Autodesk Fusion 360 part; units mm, degrees
note: some values were not read from the file. Chosen so that the rebuilt part matches the saved one: which pieces of a blend or face edit are solid.
(part 4 of 5)
  point P179 (230.75, -311.3333)
  point P180 (242.5, -311.3333)
  point P181 (242.5, -311.3333)
  point P182 (219, -320.5)
  point P183 (219, -320.5)
  point P184 (230.75, -320.5)
  point P185 (230.75, -320.5)
  point P186 (242.5, -320.5)
  point P187 (242.5, -320.5)
  point P188 (219, -265.5)
  point P189 (219, -265.5)
  point P190 (230.75, -265.5)
  point P191 (230.75, -265.5)
  point P192 (-15.5, -7.5)
  point P193 (265.5, -242.5)
  point P194 (276.5, -242.5)
  point P195 (265.5, -229.4444)
  point P196 (276.5, -229.4444)
  point P197 (287.5, -242.5)
  point P198 (298.5, -242.5)
  point P199 (309.5, -242.5)
  point P200 (287.5, -229.4444)
  point P201 (298.5, -229.4444)
  point P202 (309.5, -229.4444)
  point P203 (265.5, -216.3889)
  point P204 (276.5, -216.3889)
  point P205 (287.5, -216.3889)
  point P206 (298.5, -216.3889)
  point P207 (309.5, -216.3889)
  point P208 (265.5, -203.3333)
  point P209 (276.5, -203.3333)
  point P210 (287.5, -203.3333)
  point P211 (298.5, -203.3333)
  point P212 (309.5, -203.3333)
  point P213 (265.5, -190.2778)
  point P214 (276.5, -190.2778)
  point P215 (287.5, -190.2778)
  point P216 (298.5, -190.2778)
  point P217 (309.5, -190.2778)
  point P218 (265.5, -177.2222)
  point P219 (265.5, -164.1667)
  point P220 (276.5, -164.1667)
  point P221 (287.5, -164.1667)
  point P222 (298.5, -164.1667)
  point P223 (309.5, -164.1667)
  point P224 (265.5, -151.1111)
  point P225 (276.5, -151.1111)
  point P226 (287.5, -151.1111)
  point P227 (298.5, -151.1111)
  point P228 (309.5, -151.1111)
  point P229 (265.5, -138.0556)
  point P230 (276.5, -138.0556)
  point P231 (287.5, -138.0556)
  point P232 (298.5, -138.0556)
  point P233 (309.5, -138.0556)
  point P234 (265.5, -125)
  point P235 (276.5, -125)
  point P236 (287.5, -125)
  point P237 (298.5, -125)
  point P238 (309.5, -125)
  point P239 (265.5, -111.9444)
  point P240 (276.5, -111.9444)
  point P241 (287.5, -111.9444)
  point P242 (298.5, -111.9444)
  point P243 (309.5, -111.9444)
  point P244 (265.5, -98.8889)
  point P245 (276.5, -98.8889)
  point P246 (287.5, -98.8889)
  point P247 (298.5, -98.8889)
  point P248 (309.5, -98.8889)
  point P249 (265.5, -85.8333)
  point P250 (276.5, -85.8333)
  point P251 (287.5, -85.8333)
  point P252 (298.5, -85.8333)
  point P253 (309.5, -85.8333)
  point P254 (265.5, -72.7778)
  point P255 (276.5, -72.7778)
  point P256 (287.5, -72.7778)
  point P257 (298.5, -72.7778)
  point P258 (309.5, -72.7778)
  point P259 (265.5, -59.7222)
  point P260 (276.5, -59.7222)
  point P261 (287.5, -59.7222)
  point P262 (298.5, -59.7222)
  point P263 (309.5, -59.7222)
  point P264 (265.5, -46.6667)
  point P265 (276.5, -46.6667)
  point P266 (287.5, -46.6667)
  point P267 (298.5, -46.6667)
  point P268 (309.5, -46.6667)
  point P269 (265.5, -33.6111)
  point P270 (276.5, -33.6111)
  point P271 (287.5, -33.6111)
  point P272 (298.5, -33.6111)
  point P273 (309.5, -33.6111)
  point P274 (320.5, -242.5)
  point P275 (320.5, -229.4444)
  point P276 (320.5, -216.3889)
  point P277 (320.5, -203.3333)
  point P278 (320.5, -190.2778)
  point P279 (320.5, -177.2222)
  point P280 (320.5, -164.1667)
  point P281 (320.5, -151.1111)
  point P282 (320.5, -138.0556)
  point P283 (320.5, -125)
  point P284 (320.5, -111.9444)
  point P285 (320.5, -98.8889)
  point P286 (320.5, -85.8333)
  point P287 (320.5, -72.7778)
  point P288 (320.5, -59.7222)
  point P289 (320.5, -46.6667)
  point P290 (320.5, -33.6111)
  point P291 (265.5, -20.5556)
  point P292 (276.5, -20.5556)
  point P293 (287.5, -20.5556)
  point P294 (298.5, -20.5556)
  point P295 (309.5, -20.5556)
  point P296 (320.5, -20.5556)
  point P297 (265.5, -7.5)
  point P298 (276.5, -7.5)
  point P299 (287.5, -7.5)
  point P300 (298.5, -7.5)
  point P301 (309.5, -7.5)
  point P302 (320.5, -7.5)
  point P303 (7.6004, 372.3881)
  point P304 (250, 0)
  point P305 (240, 0)
  point P306 (432.9679, -6)
  point P307 (670.9679, -244)
  dimension "d117" = 241
  dimension "d118" = 241
  dimension "d122" = 235
  dimension "d127" = 4.5
  dimension "d128" = 4.5
  dimension "d179" = 7.5
  dimension "d418" = 8
  dimension "d420" = 11.5
  dimension "d421" = 13
  dimension "d423" = 16.5
  dimension "d425" = 13.5
  dimension "d428" = 7
  dimension "d429" = 15
  dimension "d430" = 7
  dimension "d431" = 13
  dimension "d438" = 8
  dimension "d447" = 17.5
  dimension "d451" = 20
  dimension "d457" = 8
  dimension "d458" = 7.5
  dimension "d461" = 235
  dimension "d517" = 235
  dimension "d521" = 250
  dimension "d522" = 0
  dimension "d531" = 8
  dimension "d532" = 8
  dimension "d533" = 10
  dimension "d534" = 10
  dimension "d537" = 7.5
  dimension "d538" = 7.5
  dimension "d543" = 8
  dimension "d546" = 230
  dimension "d611" = 75
  dimension "d613" = 3.5
  dimension "d614" = 16
  dimension "d616" = 15
  dimension "d617" = 6.5
  dimension "d619" = 15
  dimension "d620" = 1.75
  dimension "d621" = 1.75
  dimension "d622" = 3.75
  dimension "d623" = 3.75
  dimension "d626" = 4.5
  dimension "d627" = 4.5
  dimension "d633" = 235
  dimension "d634" = -55
  dimension "d664" = 6
  dimension "d665" = 12
  dimension "d667" = 4
  dimension "d669" = 6
  dimension "d671" = 4
  dimension "d672" = 2
  dimension "d673" = 24
  dimension "d679" = 12.5
  dimension "d791" = 4.5
  dimension "d792" = 9
  dimension "d793" = 9
  dimension "d796" = 55
  dimension "d797" = 235
  dimension "d802" = 12
  dimension "d808" = 250
  dimension "d822" = 244
  dimension "d823" = 244
  dimension "d898" = 4.5
  dimension "d899" = 3
  dimension "d904" = 3
  dimension "d919" = 0
  dimension "d939" = 3
  dimension "d940" = 3
  dimension "d1030" = 8
  constraint horizontal L3
  constraint vertical L0
  constraint coincident L0.end L3.start
  constraint vertical L1
  constraint vertical L2
  constraint horizontal L5
  constraint horizontal L6
  constraint vertical L7
  constraint coincident P0 A0.centre
  constraint equal A0 A1
  constraint coincident L2.start L8.end
  constraint horizontal L59
  constraint vertical L9
  constraint horizontal L80
  constraint vertical L10
  constraint horizontal L57
  constraint equal L14 L18
  constraint equal L13 L17
  constraint collinear L12 L16
  constraint coincident L32 L33.start
  constraint horizontal L32
  constraint vertical L48
  constraint horizontal L49
  constraint horizontal L50
  constraint vertical L199
  constraint horizontal L51
  constraint collinear L52 L59
  constraint collinear L53 L57
  constraint collinear L54 L59
  constraint collinear L55 L57
  constraint collinear L56 L59
  constraint collinear L57 L58
  constraint collinear L59 L60
  constraint vertical L79
  constraint vertical L62
  constraint horizontal L74
  constraint vertical L73
  constraint horizontal L61
  constraint vertical L72
  constraint horizontal L76
  constraint horizontal L158
  constraint vertical L75
  constraint coincident L75.start L76.end
  constraint equal L77 L78
  constraint horizontal L151
  constraint vertical L70
  constraint horizontal L78
  constraint horizontal L77
  constraint equal L62 L73
  constraint collinear L10 L75
  constraint collinear L48 L72
  constraint collinear L80 L81
  constraint horizontal L84
  constraint vertical L86
  constraint horizontal L85
  constraint vertical L87
  constraint horizontal L89
  constraint vertical L83
  constraint horizontal L82
  constraint vertical L88
  constraint equal A51 A52
  constraint coincident P2 A51.centre
  constraint horizontal L90
  constraint vertical L91
  constraint horizontal L100
  constraint vertical L103
  constraint horizontal L131
  constraint vertical L129
  constraint equal A56 A57
  constraint vertical A56.centre A57.centre
  constraint horizontal L92
  constraint vertical L93
  constraint horizontal L94
  constraint vertical L95
  constraint equal A0 A5
  constraint equal A2 A10
  constraint equal A148 A149
  constraint coincident P192 A148.centre
  constraint collinear L5 L90
  constraint collinear L100 L101
  constraint collinear L102 L129
  constraint collinear L103 L105
  constraint collinear L104 L129
  constraint collinear L105 L107
  constraint collinear L106 L129
  constraint collinear L107 L137
  constraint collinear L108 L129
  constraint coincident L119.start L137
  constraint coincident L117.start L137
  constraint coincident L110.start L137
  constraint coincident L114.start L137
  constraint coincident L112.start L137
  constraint coincident L113.end L131
  constraint coincident L115.end L129
  constraint coincident L116.end L129
  constraint coincident L118.end L129
  constraint coincident L109.end L129
  constraint collinear L126 L129
  constraint collinear L127 L129
  constraint collinear L128 L129
  constraint collinear L129 L130
  constraint collinear L131 L132
  constraint collinear L133 L137
  constraint collinear L134 L137
  constraint collinear L135 L137
  constraint collinear L136 L137
  constraint collinear L137 L138
  constraint equal A153 A154
  constraint coincident P193 A153.centre
  constraint horizontal L142
  constraint vertical L143
  constraint horizontal L144
  constraint vertical L145
  constraint horizontal L146
  constraint vertical L147
  constraint horizontal L148
  constraint vertical L149
  constraint collinear L151 L152
  constraint collinear L152 L153
  constraint collinear L153 L154
  constraint collinear L155 L158
  constraint collinear L156 L158
  constraint collinear L157 L158
  constraint collinear L158 L159
  constraint coincident L50.start L52.end
  constraint coincident P303 A10.centre
  constraint coincident P304 L1.start
  constraint coincident P305 L9.end
  constraint horizontal L160
  constraint vertical L161
  constraint horizontal L162
  constraint vertical L163
  constraint horizontal L164
  constraint vertical L165
  constraint horizontal L166
  constraint vertical L167
  constraint coincident P306 L164.start
  constraint coincident P307 L165.end
  constraint horizontal L171
  constraint vertical L170
  constraint horizontal L173
  constraint vertical L174
  constraint horizontal L175
  constraint vertical L176
  constraint collinear L11 L176
  constraint collinear L37 L174
  constraint collinear L38 L179
  constraint collinear L40 L183
  constraint collinear L43 L186
  constraint collinear L42 L187
  constraint collinear L41 L182
  constraint collinear L39 L178
  constraint collinear L173 L180
  constraint collinear L180 L184
  constraint collinear L184 L188
  constraint equal L176 L179
  constraint equal L176 L178
  constraint equal L176 L182
  constraint equal L176 L183
  constraint equal L176 L187
  constraint equal L176 L186
  constraint equal L75 L79
  constraint collinear L198 L199
  constraint collinear L199 L200
  constraint collinear L200 L201
  constraint collinear L201 L202
  constraint collinear L203 L204
  constraint collinear L204 L205
  constraint collinear L205 L206
  constraint horizontal L211
  constraint vertical L226
  constraint vertical L220
  constraint collinear L220 L222
  constraint collinear L221 L222
  constraint collinear L222 L223
  constraint collinear L224 L226
  constraint collinear L224 L225
  constraint collinear L226 L227
  constraint collinear L227 L228
  measures "d117" distance of L5.start L6.end
  measures "d118" distance of L5.start L5.end
  measures "d127" horizontal distance of L5.start L0.end
  measures "d128" vertical distance of L5.start L0.end
  measures "d179" vertical distance of L4.start A2.centre
  measures "d418" distance of L4.start L11.start
  measures "d420" distance of L28.start L28.end
  measures "d421" distance of L28.start L30.end
  measures "d423" distance of L25.end L26.end
  measures "d425" distance of L24.start L24.end
  measures "d428" distance of L20.end L21.end
  measures "d429" distance of L21.end L22.end
  measures "d430" distance of L16.end L17.end
  measures "d431" distance of L17.end L18.end
  measures "d438" diameter of A3
  measures "d447" distance of L33.start L35.end
  measures "d451" vertical distance of L4.start L32.end
  measures "d457" distance of L50.start L50.end
  measures "d458" horizontal distance of L4.end A2.centre
  measures "d531" distance of L73.start L73.end
  measures "d532" distance of L61.start L61.end
  measures "d533" distance of L61.start L78.start
  measures "d534" distance of L78.start L73.end
  measures "d537" vertical distance of L78.start P303
  measures "d538" horizontal distance of L78.start P303
  measures "d543" distance of L70.start L70.end
  measures "d546" distance of L62.end L73.start
  measures "d613" diameter of A47
  measures "d614" diameter of A48
  measures "d616" vertical distance of A48.centre A46.centre
  measures "d617" diameter of A49
  measures "d619" vertical distance of A47.centre A49.centre
  measures "d620" horizontal distance of A47.centre L84.start
  measures "d621" horizontal distance of L85.start A45.centre
  measures "d622" vertical distance of L85.start A45.centre
  measures "d623" vertical distance of A47.centre L84.start
  measures "d626" horizontal distance of L82.start P1
  measures "d627" vertical distance of L82.start P1
  measures "d664" diameter of A57
  measures "d665" vertical distance of A56.centre A57.centre
  measures "d667" vertical distance of A57.centre P10
  measures "d669" distance of L6 L94
  measures "d671" distance of A57.centre L93
  measures "d672" distance of L93 L95
  measures "d673" distance of L92 L94
  measures "d679" distance of L89 L97
  measures "d791" distance of L91 L99
  measures "d792" distance of L91 L129
  measures "d793" distance of L90 L100
  measures "d802" distance of L146.start L148.end
  measures "d808" distance of L78.start L70.start
  measures "d822" distance of L160.start L160.end
  measures "d823" distance of L160.start L162.end
  measures "d898" distance of L171 L172
  measures "d899" distance of L173.start L175.end
  measures "d904" vertical distance of L64.start L173.start
  measures "d939" distance of L163 L208
  measures "d940" distance of L160 L209
  measures "d1030" distance of L48.start L210.end
sketch "Skizze3" plane through (0, 0, 0) normal (0, 0, 1) x (1, 0, 0)
  circle A0 centre (7.5, -7.5) radius 1.5
  circle A1 centre (7.5, -7.5) radius 1.5
  line L0 (0, 0) -> (15, 0)
  line L1 (15, 0) -> (15, -15)
  line L2 (15, -15) -> (0, -15)
  line L3 (0, -15) -> (0, 0)
  line L4 (15, -15) -> (-13, -15)
  line L5 (-13, -15) -> (-13, 13)
  line L6 (-13, 13) -> (15, 13)
  line L7 (15, 13) -> (15, -15)
  line L8 (15, -15) -> (-8, -15)
  line L9 (-8, -15) -> (-8, 8)
  line L10 (-8, 8) -> (15, 8)
  line L11 (15, 8) -> (15, -15)
  line L12 (-8, -15) -> (-11, -15)
  line L13 (-11, -15) -> (-11, -4.5)
  line L14 (-11, -4.5) -> (-8, -4.5)
  line L15 (-8, -4.5) -> (-8, -15)
  line L16 (15, 8) -> (4.5, 8)
  line L17 (4.5, 11) -> (15, 11)
  line L18 (15, 11) -> (15, 8)
  line L19 (0, 0) -> (10.8258, 0)
  line L20 (10.8258, 0) -> (10.8258, 2.5)
  line L21 (10.8258, 2.5) -> (0, 2.5)
  line L22 (0, 2.5) -> (0, 0)
  line L23 (0, 2.5) -> (15, 2.5)
  line L24 (15, 2.5) -> (15, 5.5)
  line L25 (15, 5.5) -> (0, 5.5)
  line L26 (0, 5.5) -> (0, 2.5)
  line L27 (29.799, -19.957) -> (29.799, -30.0096)
  line L28 (24.9821, -24.9833) -> (34.8253, -24.9833)
  line L29 (4.5, -4.5) -> (15, -4.5)
  line L30 (15, -4.5) -> (15, -15)
  line L31 (15, -15) -> (4.5, -15)
  line L32 (4.5, -15) -> (4.5, -4.5)
  line L33 (4.5, 8) -> (4.5, 11)
  line L34 (4.5, -4.5) -> (245.5, -4.5)
  line L35 (0, 5.5) -> (0, 8)
  line L36 (44.598, -15) -> (59.598, -15)
  line L37 (59.598, 2.5) -> (44.598, 2.5)
  line L38 (48.7722, 0) -> (48.7722, 2.5)
  line L39 (59.598, -15) -> (59.598, 0)
  line L40 (59.598, 0) -> (48.7722, 0)
  line L41 (67.598, -4.5) -> (67.598, -15)
  line L42 (72.598, 13) -> (44.598, 13)
  line L43 (55.098, 11) -> (44.598, 11)
  line L44 (72.598, -15) -> (72.598, 13)
  line L45 (67.598, -15) -> (70.598, -15)
  line L46 (59.598, 5.5) -> (59.598, 8)
  line L47 (44.598, 5.5) -> (59.598, 5.5)
  line L48 (44.598, 0) -> (44.598, -15)
  line L49 (55.098, 8) -> (55.098, 11)
  line L50 (44.598, 8) -> (44.598, -15)
  line L51 (70.598, -4.5) -> (67.598, -4.5)
  line L52 (44.598, -15) -> (67.598, -15)
  line L53 (67.598, 8) -> (44.598, 8)
  circle A2 centre (52.098, -7.5) radius 1.5
  line L54 (44.598, -15) -> (55.098, -15)
  line L55 (67.598, -15) -> (67.598, 8)
  line L56 (44.598, 11) -> (44.598, 8)
  line L57 (44.598, -4.5) -> (44.598, -15)
  line L58 (44.598, 2.5) -> (44.598, 5.5)
  line L59 (59.598, 2.5) -> (59.598, 0)
  circle A3 centre (52.098, -7.5) radius 1.5
  line L60 (70.598, -15) -> (70.598, -4.5)
  line L61 (55.098, -15) -> (55.098, -4.5)
  line L62 (59.598, 5.5) -> (59.598, 2.5)
  line L63 (55.098, -4.5) -> (44.598, -4.5)
  line L64 (44.598, -15) -> (72.598, -15)
  line L65 (48.7722, 2.5) -> (59.598, 2.5)
  line L66 (59.598, 0) -> (44.598, 0)
  line L67 (44.598, 8) -> (55.098, 8)
  line L68 (44.598, 13) -> (44.598, -15)
  line L69 (15, -52.4665) -> (15, -55.4665)
  line L70 (44.598, -49.9665) -> (44.598, -34.9665)
  line L71 (48.7722, -49.9665) -> (48.7722, -52.4665)
  circle A4 centre (52.098, -42.4665) radius 1.5
  line L72 (44.598, -45.4665) -> (44.598, -34.9665)
  circle A5 centre (52.098, -42.4665) radius 1.5
  line L73 (59.598, -49.9665) -> (44.598, -49.9665)
  line L74 (59.598, -52.4665) -> (44.598, -52.4665)
  line L75 (44.598, -34.9665) -> (59.598, -34.9665)
  line L76 (44.598, -34.9665) -> (67.598, -34.9665)
  line L77 (55.098, -60.9665) -> (44.598, -60.9665)
  line L78 (55.098, -45.4665) -> (44.598, -45.4665)
  line L79 (67.598, -57.9665) -> (44.598, -57.9665)
  line L80 (59.598, -49.9665) -> (48.7722, -49.9665)
  line L81 (48.7722, -52.4665) -> (59.598, -52.4665)
  line L82 (44.598, -34.9665) -> (72.598, -34.9665)
  line L83 (72.598, -62.9665) -> (44.598, -62.9665)
  line L84 (44.598, -57.9665) -> (55.098, -57.9665)
  line L85 (44.598, -55.4665) -> (59.598, -55.4665)
  line L86 (44.598, -34.9665) -> (55.098, -34.9665)
  line L87 (15, -45.4665) -> (15, -34.9665)
  line L88 (4.5, -34.9665) -> (4.5, -45.4665)
  line L89 (15, -57.9665) -> (15, -34.9665)
  line L90 (-8, -34.9665) -> (-8, -57.9665)
  line L91 (-8, -57.9665) -> (15, -57.9665)
  line L92 (44.598, -62.9665) -> (44.598, -34.9665)
  line L93 (10.8258, -52.4665) -> (0, -52.4665)
  line L94 (0, -55.4665) -> (0, -57.9665)
  line L95 (15, -57.9665) -> (4.5, -57.9665)
  line L96 (0, -52.4665) -> (15, -52.4665)
  line L97 (0, -49.9665) -> (10.8258, -49.9665)
  line L98 (44.598, -60.9665) -> (44.598, -57.9665)
  line L99 (15, -62.9665) -> (15, -34.9665)
  line L100 (44.598, -52.4665) -> (44.598, -55.4665)
  line L101 (15, -34.9665) -> (0, -34.9665)
  line L102 (15, -60.9665) -> (15, -57.9665)
  line L103 (-13, -34.9665) -> (-13, -62.9665)
  circle A6 centre (7.5, -42.4665) radius 1.5
  line L104 (-11, -45.4665) -> (-8, -45.4665)
  line L105 (0, -49.9665) -> (15, -49.9665)
  line L106 (4.5, -57.9665) -> (4.5, -60.9665)
  line L107 (44.598, -57.9665) -> (44.598, -34.9665)
  line L108 (0, -52.4665) -> (0, -49.9665)
  line L109 (0, -34.9665) -> (0, -49.9665)
  line L110 (10.8258, -49.9665) -> (10.8258, -52.4665)
  line L111 (0, -55.4665) -> (0, -52.4665)
  circle A7 centre (7.5, -42.4665) radius 1.5
  line L112 (4.5, -45.4665) -> (15, -45.4665)
  line L113 (15, -34.9665) -> (-13, -34.9665)
  line L114 (15, -49.9665) -> (15, -34.9665)
  line L115 (15, -34.9665) -> (4.5, -34.9665)
  line L116 (15, -55.4665) -> (0, -55.4665)
  line L117 (4.5, -60.9665) -> (15, -60.9665)
  line L118 (-8, -34.9665) -> (-11, -34.9665)
  line L119 (-13, -62.9665) -> (15, -62.9665)
  line L120 (-8, -45.4665) -> (-8, -34.9665)
  line L121 (-11, -34.9665) -> (-11, -45.4665)
  line L122 (15, -34.9665) -> (-8, -34.9665)
  line L123 (59.598, -52.4665) -> (59.598, -49.9665)
  line L124 (59.598, -55.4665) -> (59.598, -57.9665)
  line L125 (70.598, -34.9665) -> (70.598, -45.4665)
  line L126 (67.598, -34.9665) -> (67.598, -57.9665)
  line L127 (67.598, -45.4665) -> (67.598, -34.9665)
  line L128 (59.598, -55.4665) -> (59.598, -52.4665)
  line L129 (59.598, -34.9665) -> (59.598, -49.9665)
  line L130 (55.098, -57.9665) -> (55.098, -60.9665)
  line L131 (55.098, -34.9665) -> (55.098, -45.4665)
  line L132 (70.598, -45.4665) -> (67.598, -45.4665)
  line L133 (72.598, -34.9665) -> (72.598, -62.9665)
  line L134 (67.598, -34.9665) -> (70.598, -34.9665)
  point P0 (7.5, -7.5)
  point P1 (4.5, -4.5)
  point P2 (59.598, 0)
  point P3 (52.098, -7.5)
  point P4 (55.098, -4.5)
  point P5 (55.098, -4.5)
  point P6 (7.5, -42.4665)
  point P7 (55.098, -45.4665)
  point P8 (52.098, -42.4665)
  point P9 (55.098, -45.4665)
  point P10 (0, -49.9665)
  point P11 (59.598, -49.9665)
  point P12 (4.5, -45.4665)
  point P13 (4.5, -45.4665)
  dimension "d971" = 15
  dimension "d972" = 15
  dimension "d973" = 28
  dimension "d974" = 28
  dimension "d975" = 23
  dimension "d976" = 23
  dimension "d977" = 3
  dimension "d980" = 3
  dimension "d981" = 2.5
  dimension "d982" = 3
  constraint coincident P0 A0.centre
  constraint equal A0 A1
  constraint horizontal L0
  constraint vertical L1
  constraint horizontal L2
  constraint vertical L3
  constraint coincident L0.start L3.end
  constraint horizontal L4
  constraint vertical L5
  constraint horizontal L6
  constraint vertical L7
  constraint horizontal L8
  constraint vertical L9
  constraint horizontal L10
  constraint vertical L11
  constraint horizontal L12
  constraint vertical L13
  constraint horizontal L14
  constraint vertical L15
  constraint horizontal L16
  constraint horizontal L17
  constraint vertical L18
  constraint horizontal L19
  constraint vertical L20
  constraint horizontal L21
  constraint vertical L22
  constraint horizontal L23
  constraint vertical L24
  constraint horizontal L25
  constraint vertical L26
  constraint coincident L7 L24.end
  constraint vertical L27
  constraint perpendicular L27 L28
  constraint horizontal L29
  constraint vertical L30
  constraint horizontal L31
  constraint vertical L32
  constraint coincident P1 L29.start
  constraint perpendicular L17 L33
  constraint collinear L32 L33
  constraint collinear L14 L34
  constraint coincident L10 L35.end
  constraint perpendicular L10 L35
  constraint symmetric L0.start L27 P2
  constraint symmetric A0 L27 A2
  constraint symmetric P0 L27 P3
  constraint symmetric A1 L27 A3
  constraint symmetric L0.end L27 L48.start
  constraint symmetric L1.end L27 L36.start
  constraint symmetric L2.end L27 L36.end
  constraint symmetric L4.end L27 L44.start
  constraint symmetric L5.end L27 L42.start
  constraint symmetric L6.end L27 L42.end
  constraint symmetric L8.end L27 L41.end
  constraint symmetric L9.end L27 L53.start
  constraint symmetric L10.end L27 L50.start
  constraint symmetric L12.end L27 L45.end
  constraint symmetric L13.end L27 L51.start
  constraint symmetric L14.end L27 L41.start
  constraint symmetric L16.end L27 L49.start
  constraint symmetric L17.start L27 L43.start
  constraint symmetric L17.end L27 L43.end
  constraint symmetric L19.end L27 L38.start
  constraint symmetric L20.end L27 L38.end
  constraint symmetric L21.end L27 L37.start
  constraint symmetric L23.end L27 L37.end
  constraint symmetric L24.end L27 L47.start
  constraint symmetric L25.end L27 L46.start
  constraint symmetric L27 P1 P5
  constraint symmetric L27 L29.end L57.start
  constraint symmetric L27 L31.end L54.end
  constraint symmetric L27 L35.end L46.end
  constraint symmetric L0.start L28 P10
  constraint symmetric A0 L28 A7
  constraint symmetric P0 L28 P6
  constraint symmetric A1 L28 A6
  constraint symmetric L0.end L28 L105.end
  constraint symmetric L1.end L28 L87.end
  constraint symmetric L2.end L28 L101.end
  constraint symmetric L4.end L28 L103.start
  constraint symmetric L5.end L28 L103.end
  constraint symmetric L6.end L28 L99.start
  constraint symmetric L8.end L28 L90.start
  constraint symmetric L9.end L28 L90.end
  constraint symmetric L10.end L28 L89.start
  constraint symmetric L12.end L28 L118.end
  constraint symmetric L13.end L28 L104.start
  constraint symmetric L14.end L28 L104.end
  constraint symmetric L16.end L28 L95.end
  constraint symmetric L17.start L28 L106.end
  constraint symmetric L17.end L28 L102.start
  constraint symmetric L19.end L28 L97.end
  constraint symmetric L20.end L28 L93.start
  constraint symmetric L21.end L28 L93.end
  constraint symmetric L23.end L28 L69.start
  constraint symmetric L24.end L28 L69.end
  constraint symmetric L25.end L28 L94.start
  constraint symmetric L28 P1 P13
  constraint symmetric L28 L29.end L87.start
  constraint symmetric L28 L31.end L88.start
  constraint symmetric L28 L35.end L94.end
  constraint symmetric L28 L37.start L74.start
  constraint symmetric L28 L36.end L75.end
  constraint symmetric L28 L41.end L76.end
  constraint symmetric L28 L54.end L86.end
  constraint symmetric L28 L38.start L71.start
  constraint symmetric L28 L46.start L85.end
  constraint symmetric L28 L48.start L70.start
  constraint symmetric L28 L46.end L124.end
  constraint symmetric L28 L36.start L70.end
  constraint symmetric L28 L42.start L83.start
  constraint symmetric L28 P2 P11
  constraint symmetric L28 L50.start L79.end
  constraint symmetric L28 L42.end L83.end
  constraint symmetric L28 L45.end L125.start
  constraint symmetric L28 P3 P8
  constraint symmetric L28 L57.start L72.start
  constraint symmetric L28 L41.start L127.start
  constraint symmetric L28 P5 P9
  constraint symmetric L28 L51.start L125.end
  constraint symmetric L28 L49.start L84.end
  constraint symmetric L28 L43.start L77.start
  constraint symmetric L28 L37.end L74.end
  constraint symmetric L28 L53.start L79.start
  constraint symmetric L28 L47.start L85.start
  constraint symmetric L28 L44.start L82.end
  constraint symmetric L28 L38.end L71.end
  constraint symmetric L28 L43.end L77.end
  constraint symmetric L28 A2 A5
  constraint symmetric L28 A3 A4
  measures "d971" distance of L0.start L0.end
  measures "d972" distance of L0.start L2.end
  measures "d973" distance of L1.end L4.end
  measures "d974" distance of L1.end L6.end
  measures "d975" distance of L1.end L8.end
  measures "d976" distance of L1.end L10.end
  measures "d977" distance of L8.end L12.end
  measures "d980" distance of L10.end L17.end
  measures "d981" distance of L0.start L21.end
  measures "d982" distance of L21.end L25.end
sketch "Skizze4" plane through (-10, 0, 0) normal (-1, 0, 0) x (0, -1, 0)
  line L0 (-10, 0) -> (-8, 0)
  line L1 (15, 70) -> (15, 75)
  line L2 (15, 75) -> (-10, 75)
  line L3 (-10, 75) -> (-10, 0)
  circle A0 centre (7.5, 62.5) radius 1.5
  circle A1 centre (7.5, 7.5) radius 1.5
  line L4 (-8, 70) -> (15, 70)
  line L5 (-8, 0) -> (-8, 70)
  point P0 (-10, 0)
  dimension "d167" = 3
  dimension "d168" = 17.5
  dimension "d169" = 12.5
  dimension "d337" = 3
  dimension "d338" = 17.5
  dimension "d339" = 7.5
  measures "d167" diameter of A0
  measures "d168" horizontal distance of L2.end A0.centre
  measures "d169" vertical distance of L2.end A0.centre
  measures "d337" diameter of A1
  measures "d338" horizontal distance of A1.centre P0
  measures "d339" vertical distance of A1.centre origin
sketch "Skizze5" plane through (0, 0, 0) normal (0, 0, 1) x (1, 0, 0)
  line L0 (0, 7.8901) -> (0, 0)
  line L1 (15, 20) -> (40, 20)
  line L2 (40, 20) -> (40, 45)
  line L3 (40, 45) -> (15, 45)
  line L4 (15, 45) -> (15, 20)
  line L5 (40, 45) -> (17, 45)
  line L6 (17, 45) -> (17, 22)
  line L7 (17, 22) -> (40, 22)
  line L8 (40, 22) -> (40, 45)
  circle A0 centre (32.5, 37.5) radius 1.5
  dimension "d207" = 25
  dimension "d208" = 23
  dimension "d209" = 3
  dimension "d210" = 7.5
  dimension "d211" = 7.5
  constraint horizontal L1
  constraint vertical L2
  constraint horizontal L3
  constraint vertical L4
  constraint equal L1 L4
  constraint horizontal L5
  constraint vertical L6
  constraint horizontal L7
  constraint vertical L8
  constraint equal L5 L8
  measures "d207" distance of L1.start L3.end
  measures "d208" distance of L2.end L7.end
  measures "d209" diameter of A0
  measures "d210" horizontal distance of L2.end A0.centre
  measures "d211" vertical distance of L2.end A0.centre
sketch "Skizze6" plane through (0, 0, 0) normal (0, 0, 1) x (1, 0, 0)
  line L0 (45.0336, 39.9327) -> (60.0336, 39.9327)
  line L1 (60.0336, 39.9327) -> (60.0336, 24.9327)
  line L2 (60.0336, 24.9327) -> (45.0336, 24.9327)
  line L3 (45.0336, 24.9327) -> (45.0336, 39.9327)
  line L4 (60.0336, 39.9327) -> (47.0336, 39.9327)
  line L5 (47.0336, 39.9327) -> (47.0336, 26.9327)
  line L6 (47.0336, 26.9327) -> (60.0336, 26.9327)
  line L7 (60.0336, 26.9327) -> (60.0336, 39.9327)
  circle A0 centre (52.5336, 32.4327) radius 1.5
  dimension "d213" = 15
  dimension "d214" = 13
  dimension "d243" = 3
  dimension "d244" = 7.5
  dimension "d245" = 7.5
  constraint horizontal L0
  constraint vertical L1
  constraint horizontal L2
  constraint vertical L3
  constraint equal L0 L3
  constraint horizontal L4
  constraint vertical L5
  constraint horizontal L6
  constraint vertical L7
  constraint equal L5 L6
  measures "d213" distance of L0.start L2.end
  measures "d214" distance of L0.end L6.end
  measures "d243" diameter of A0
  measures "d244" horizontal distance of L0.end A0.centre
  measures "d245" vertical distance of L0.end A0.centre
extrude "Extrusion7" add sketch "Skizze5" along normal blind 2 contours L2 L3 L5 L6 L7 L8 makes body 1
extrude "Extrusion8" add sketch "Skizze6" along normal blind 2 separate body contours L0 L1 L4 L5 L6 L7 | A0 makes body 2
extrude "Extrusion9" add sketch "Skizze5" along normal blind 25 contours L1 L2 L3 L4 L6 L7 bodies 1
extrude "Extrusion10" add sketch "Skizze6" along normal blind 15 contours L0 L1 L2 L3 L5 L6 bodies 2
sketch "Skizze7" plane through (0, 24.9327, 0) normal (0, -1, 0) x (1, 0, 0)
  line L0 (45.0336, 0) -> (60.0336, 0)
  line L1 (60.0336, 0) -> (60.0336, 15)
  line L2 (60.0336, 15) -> (45.0336, 15)
  line L3 (45.0336, 15) -> (45.0336, 0)
  circle A0 centre (52.5336, 7.5) radius 1.5
  dimension "d223" = 3
  dimension "d224" = 7.5
  dimension "d225" = 7.5
  measures "d223" diameter of A0
  measures "d224" horizontal distance of L1.end A0.centre
  measures "d225" vertical distance of L1.end A0.centre
sketch "Skizze8" plane through (0, 20, 0) normal (0, -1, 0) x (1, 0, 0)
  line L0 (15, 0) -> (40, 0)
  line L1 (40, 0) -> (40, 25)
  line L2 (40, 25) -> (15, 25)
  line L3 (15, 25) -> (15, 0)
  circle A0 centre (32.5, 17.5) radius 1.5
  dimension "d226" = 3
  dimension "d227" = 7.5
  dimension "d228" = 7.5
  measures "d226" diameter of A0
  measures "d227" horizontal distance of L1.end A0.centre
  measures "d228" vertical distance of L1.end A0.centre
sketch "Skizze9" plane through (15, 0, 0) normal (-1, 0, 0) x (0, -1, 0)
  line L0 (-45, 0) -> (-20, 0)
  line L1 (-20, 0) -> (-20, 25)
  line L2 (-20, 25) -> (-45, 25)
  line L3 (-45, 25) -> (-45, 0)
  circle A0 centre (-37.5, 17.5) radius 1.5
  dimension "d229" = 3
  dimension "d230" = 7.5
  dimension "d231" = 7.5
  measures "d229" diameter of A0
  measures "d230" vertical distance of L2.end A0.centre
  measures "d231" horizontal distance of L2.end A0.centre
sketch "Skizze10" plane through (45.0336, 0, 0) normal (-1, 0, 0) x (0, -1, 0)
  line L0 (-39.9327, 0) -> (-24.9327, 0)
  line L1 (-24.9327, 0) -> (-24.9327, 15)
  line L2 (-24.9327, 15) -> (-39.9327, 15)
  line L3 (-39.9327, 15) -> (-39.9327, 0)
  circle A0 centre (-32.4327, 7.5) radius 1.5
  dimension "d232" = 3
  dimension "d233" = 7.5
  dimension "d234" = 7.5
  measures "d232" diameter of A0
  measures "d233" horizontal distance of L2.end A0.centre
  measures "d234" vertical distance of L2.end A0.centre
extrude "Extrusion11" cut sketch "Skizze8" against normal blind 2 contours A0 bodies 1
extrude "Extrusion12" cut sketch "Skizze9" against normal blind 2 contours A0 bodies 1
extrude "Extrusion13" cut sketch "Skizze7" against normal blind 2 contours A0 bodies 2
extrude "Extrusion14" cut sketch "Skizze10" against normal blind 2 contours A0 bodies 2
extrude "Extrusion15" cut sketch "Skizze6" along normal blind 2 contours A0 bodies 2
sketch "Skizze11" plane through (0, 0, 0) normal (0, 0, 1) x (1, 0, 0)
  line L0 (15, 50) -> (40, 50)
  line L1 (40, 50) -> (40, 65)
  line L2 (40, 65) -> (15, 65)
  line L3 (15, 65) -> (15, 50)
  line L4 (40, 65) -> (17, 65)
  line L5 (17, 65) -> (17, 50)
  line L6 (17, 50) -> (40, 50)
  line L7 (40, 50) -> (40, 65)
  circle A0 centre (32.5, 57.5) radius 1.5
  line L8 (40, 116) -> (15, 116)
  line L9 (40, 75) -> (40, 116)
  line L10 (17, 116) -> (17, 75)
  line L11 (40, 75) -> (40, 116)
  line L12 (17, 75) -> (40, 75)
  line L13 (40, 116) -> (17, 116)
  line L14 (15, 75) -> (40, 75)
  line L15 (15, 116) -> (15, 75)
  circle A1 centre (32.5, 108.5) radius 1.5
  circle A2 centre (32.5, 82.5) radius 1.5
  dimension "d301" = 25
  dimension "d302" = 15
  dimension "d303" = 23
  dimension "d304" = 3
  dimension "d305" = 7.5
  dimension "d306" = 7.5
  dimension "d1009" = 25
  dimension "d1010" = 41
  dimension "d1011" = 23
  dimension "d1012" = 3
  dimension "d1013" = 7.5
  dimension "d1014" = 7.5
  dimension "d1015" = 3
  dimension "d1016" = 7.5
  dimension "d1017" = 7.5
  constraint horizontal L0
  constraint vertical L1
  constraint horizontal L2
  constraint vertical L3
  constraint horizontal L4
  constraint vertical L5
  constraint horizontal L6
  constraint vertical L7
  constraint horizontal L14
  constraint vertical L9
  constraint horizontal L8
  constraint vertical L15
  constraint horizontal L13
  constraint vertical L10
  constraint horizontal L12
  constraint vertical L11
  measures "d301" distance of L0.start L0.end
  measures "d302" distance of L0.start L2.end
  measures "d303" distance of L1.end L4.end
  measures "d304" diameter of A0
  measures "d305" horizontal distance of L1.end A0.centre
  measures "d306" vertical distance of L1.end A0.centre
  measures "d1009" distance of L14.start L9.start
  measures "d1010" distance of L14.start L8.end
  measures "d1011" distance of L8.start L10.start
  measures "d1012" diameter of A1
  measures "d1013" horizontal distance of L8.start A1.centre
  measures "d1014" vertical distance of L8.start A1.centre
  measures "d1015" diameter of A2
  measures "d1016" distance of L11 A2.centre
  measures "d1017" distance of L14 A2.centre
extrude "Extrusion16" add sketch "Skizze11" along normal blind 2 separate body contours L0 L1 L2 L4 L5 L6 L7 | L8 L9 L10 L11 L12 L13 L14 makes body 3 at (21.6667, 57.5, 0) makes body 4 at (21.7535, 91.4483, 0)
extrude "Extrusion17" add sketch "Skizze11" along normal blind 25 contours L0 L2 L3 L5 | L8 L10 L14 L15 bodies 3 4
sketch "Skizze12" plane through (15, 0, 0) normal (-1, 0, 0) x (0, -1, 0)
  line L0 (-65, 0) -> (-50, 0)
  line L1 (-50, 0) -> (-50, 25)
  line L2 (-50, 25) -> (-65, 25)
  line L3 (-65, 25) -> (-65, 0)
  circle A0 centre (-57.5, 17.5) radius 1.5
  circle A1 centre (-108.5, 17.5) radius 1.5
  circle A2 centre (-82.5, 17.5) radius 1.5
  line L4 (-75, 0) -> (-75, 25)
  line L5 (-116, 0) -> (-116, 25)
  line L6 (-116, 25) -> (-75, 25)
  dimension "d311" = 3
  dimension "d312" = 7.5
  dimension "d313" = 7.5
  dimension "d1018" = 3
  dimension "d1019" = 3
  dimension "d1020" = 7.5
  dimension "d1021" = 7.5
  dimension "d1022" = 7.5
  dimension "d1023" = 7.5
  measures "d311" diameter of A0
  measures "d312" horizontal distance of L2.end A0.centre
  measures "d313" vertical distance of L2.end A0.centre
  measures "d1018" diameter of A1
  measures "d1019" diameter of A2
  measures "d1020" distance of A2.centre L4
  measures "d1021" distance of A1.centre L5
  measures "d1022" distance of A1.centre L6
  measures "d1023" distance of A2.centre L6
sketch "Skizze13" plane through (0, 0, 0) normal (0, 0, 1) x (1, 0, 0)
  line L0 (45.0336, 49.7292) -> (60.0336, 49.7292)
  line L1 (60.0336, 49.7292) -> (60.0336, 64.7292)
  line L2 (60.0336, 64.7292) -> (45.0336, 64.7292)
  line L3 (45.0336, 64.7292) -> (45.0336, 49.7292)
  circle A0 centre (52.5336, 57.2292) radius 1.5
  line L4 (60.0336, 64.7292) -> (47.0336, 64.7292)
  line L5 (47.0336, 64.7292) -> (47.0336, 49.7292)
  line L6 (47.0336, 49.7292) -> (60.0336, 49.7292)
  line L7 (60.0336, 49.7292) -> (60.0336, 64.7292)
  line L8 (47.0336, 62.7292) -> (60.0336, 62.7292)
  line L9 (60.0336, 62.7292) -> (60.0336, 51.7292)
  line L10 (60.0336, 51.7292) -> (47.0336, 51.7292)
  line L11 (47.0336, 51.7292) -> (47.0336, 62.7292)
  dimension "d314" = 15
  dimension "d315" = 15
  dimension "d316" = 3
  dimension "d317" = 7.5
  dimension "d318" = 7.5
  dimension "d319" = 13
  dimension "d320" = 15
  dimension "d321" = 13
  dimension "d322" = 11
  dimension "d323" = 2
  constraint horizontal L0
  constraint vertical L1
  constraint horizontal L2
  constraint vertical L3
  constraint horizontal L4
  constraint vertical L5
  constraint horizontal L6
  constraint vertical L7
  constraint horizontal L8
  constraint vertical L9
  constraint horizontal L10
  constraint vertical L11
  constraint coincident L5 L8.start
  measures "d314" distance of L0.start L0.end
  measures "d315" distance of L0.start L2.end
  measures "d316" diameter of A0
  measures "d317" horizontal distance of L1.end A0.centre
  measures "d318" vertical distance of L1.end A0.centre
  measures "d319" distance of L1.end L4.end
  measures "d320" distance of L1.end L0.end
  measures "d321" distance of L8.start L8.end
  measures "d322" distance of L8.start L10.end
  measures "d323" distance of L4.end L8.start
extrude "Extrusion18" add sketch "Skizze13" along normal blind 2 separate body contours L1 L5 L7 L8 L9 L10 L11 makes body 5
extrude "Extrusion19" add sketch "Skizze13" along normal blind 15 contours L0 L1 L5 L6 L7 L10 | L1 L2 L4 L5 L7 L8 bodies 5
extrude "Extrusion20" add sketch "Skizze13" along normal blind 15 contours L0 L2 L3 L5 L11 bodies 5
draft "Entwurf1" angle -45 neutral plane through (45.0336, 64.7292, 0) pull (-1, 0, 0) 1 faces at (50.7003, 50.3959, 15) on bodies 5
sketch "Skizze14" plane through (45.0336, 0, 0) normal (-1, 0, 0) x (0, -1, 0)
  line L0 (-64.7292, 0) -> (-49.7292, 0)
  line L1 (-49.7292, 0) -> (-49.7292, 15)
  line L2 (-49.7292, 15) -> (-64.7292, 15)
  line L3 (-64.7292, 15) -> (-64.7292, 0)
  circle A0 centre (-57.2292, 7.5) radius 1.5
  dimension "d332" = 3
  dimension "d333" = 7.5
  dimension "d334" = 7.5
  measures "d332" diameter of A0
  measures "d333" horizontal distance of L2.end A0.centre
  measures "d334" vertical distance of L2.end A0.centre
extrude "Extrusion21" cut sketch "Skizze14" against normal blind 2 contours A0 bodies 5
extrude "Extrusion23" cut sketch "Skizze12" against normal blind 2 contours A0 | A1 | A2 bodies 3 4
extrude "Extrusion24" add sketch "Skizze3" along normal blind 5 separate body contours L0 L19 L20 L21 L22 L23 | L0 L1 L2 L3 L4 L7 L8 L11 L19 L29 L32 L34 | L3 L4 L8 L9 L10 L15 L22 L26 L35 | L0 L7 L11 L20 L23 | L7 L11 L21 L23 L24 L25 L26 | L4 L9 L12 L13 L14 L15 | L7 L10 L11 L16 L25 L35 | L4 L5 L6 L7 L9 L10 L13 L14 L17 L33 | L7 L10 L16 L17 L18 L33 | L34 L39 L40 L48 L50 L63 L66 L68 | L34 L36 L39 L52 L61 L64 | L37 L38 L50 L66 L68 | L34 L39 L46 L53 L55 L59 L62 | L34 L39 L41 L52 L55 L64 | L37 L47 L50 L58 L62 L65 L68 | L37 L38 L40 L59 L65 L66 | L34 L42 L43 L44 L49 L51 L53 L55 L68 | L34 L41 L45 L51 L55 L60 L64 | L46 L47 L50 L53 L67 L68 | L34 L44 L60 L64 | L43 L49 L53 L56 L67 L68 | L89 L96 L99 L105 L110 | L69 L89 L93 L96 L99 L111 L116 | L89 L91 L94 L95 L99 L116 | L88 L89 L97 L99 L101 L105 L109 L112 L113 L114 L122 | L93 L96 L97 L105 L108 L110 | L91 L95 L99 L102 L106 L117 | L90 L91 L94 L108 L109 L111 L113 L120 L122 | L90 L91 L99 L103 L104 L106 L113 L117 L119 L121 | L90 L104 L113 L118 L120 L121 | L70 L73 L75 L76 L78 L80 L82 L92 L107 L129 L131 | L71 L73 L74 L92 L107 | L71 L73 L74 L80 L81 L123 | L74 L81 L85 L92 L100 L107 L128 | L76 L79 L82 L123 L124 L126 L127 L128 L129 | L79 L84 L85 L92 L107 L124 | L77 L79 L84 L92 L98 L130 | L82 L125 L126 L127 L132 L134 | L77 L79 L82 L83 L92 L125 L126 L130 L132 L133 makes body 6 at (-7.1667, -2.1667, 0) makes body 7 at (-7.1667, -47.7999, 5) makes body 8 at (57.4313, -57.1332, 5) makes body 9 at (57.4313, 7.1667, 0)
extrude "Extrusion32" add sketch "Skizze3" along normal blind 2 contours L1 L2 L4 L7 L8 L11 L29 L30 L31 L32 L34 | L34 L36 L48 L50 L52 L54 L57 L61 L63 L64 L68 | L87 L88 L89 L99 L101 L112 L113 L114 L115 L122 | L70 L72 L75 L76 L78 L82 L86 L92 L107 L131 bodies 7 8 6 9
extrude "Extrusion33" add sketch "Skizze3" along normal blind 28 contours L7 L10 L11 L16 L25 L35 | L4 L5 L6 L7 L9 L10 L13 L14 L17 L33 | L7 L10 L16 L17 L18 L33 | L34 L42 L43 L44 L49 L51 L53 L55 L68 | L46 L47 L50 L53 L67 L68 | L34 L44 L60 L64 | L43 L49 L53 L56 L67 L68 | L90 L91 L99 L103 L104 L106 L113 L117 L119 L121 | L77 L79 L82 L83 L92 L125 L126 L130 L132 L133 bodies 7 8 6 9
extrude "Extrusion34" add sketch "Skizze3" along normal blind 17.5 contours L4 L9 L12 L13 L14 L15 | L34 L41 L45 L51 L55 L60 L64 | L91 L95 L99 L102 L106 L117 | L90 L104 L113 L118 L120 L121 | L77 L79 L84 L92 L98 L130 | L82 L125 L126 L127 L132 L134 bodies 7 8 6 9
sketch "Skizze18" plane through (-13, 0, 0) normal (-1, 0, 0) x (0, -1, 0)
  line L0 (34.9665, 0) -> (62.9665, 0)
  line L1 (62.9665, 0) -> (62.9665, 28)
  line L2 (62.9665, 28) -> (34.9665, 28)
  line L3 (34.9665, 28) -> (34.9665, 0)
  circle A0 centre (42.4665, 20.5) radius 1.5
  circle A1 centre (7.5, 20.5) radius 1.5
  line L4 (15, 0) -> (15, 28)
  line L5 (-13, 28) -> (15, 28)
  dimension "d993" = 3
  dimension "d994" = 3
  dimension "d995" = 7.5
  dimension "d996" = 7.5
  dimension "d997" = 7.5
  dimension "d998" = 7.5
  measures "d993" diameter of A0
  measures "d994" diameter of A1
  measures "d995" distance of L3 A0.centre
  measures "d996" distance of L2 A0.centre
  measures "d997" distance of A1.centre L4
  measures "d998" distance of A1.centre L5
sketch "Skizze19" plane through (0, -62.9665, 0) normal (0, -1, 0) x (1, 0, 0)
  line L0 (44.598, 0) -> (72.598, 0)
  line L1 (72.598, 0) -> (72.598, 28)
  line L2 (72.598, 28) -> (44.598, 28)
  line L3 (44.598, 28) -> (44.598, 0)
  circle A0 centre (52.098, 20.5) radius 1.5
  circle A1 centre (7.5, 20.5) radius 1.5
  line L4 (15, 0) -> (15, 28)
  line L5 (-13, 28) -> (15, 28)
  dimension "d999" = 3
  dimension "d1000" = 3
  dimension "d1001" = 7.5
  dimension "d1002" = 7.5
  dimension "d1003" = 7.5
  dimension "d1004" = 7.5
  measures "d999" diameter of A0
  measures "d1000" diameter of A1
  measures "d1001" distance of A1.centre L4
  measures "d1002" distance of L3 A0.centre
  measures "d1003" distance of L2 A0.centre
  measures "d1004" distance of A1.centre L5
extrude "Extrusion35" cut sketch "Skizze19" against normal blind 77 contours A0 | A1 bodies 7 8 6 9
extrude "Extrusion36" cut sketch "Skizze18" against normal blind 88 contours A0 | A1 bodies 7 8 6 9
equation "box_iw = 250 mm"
equation "box_id = 250 mm"
equation "box_ih = 70 mm"
equation "screwd = 3 mm"
equation "lcd_screwd = 3.5 mm"
equation "button_screwd = 16 mm"
equation "lcd_boardw = 75 mm"
equation "lcd_boardh = 30 mm"
equation "lcd_xtl = ( box_iw - lcd_boardw - button_screwd ) / 2"
equation "lcd_ytl = ( box_ih - lcd_boardh - button_screwd ) / 2"
equation "cornerdim = 15 mm"
equation "d12 = box_iw"
equation "d13 = box_id"
equation "wallthickness = 8 mm"
equation "platethickness = 3 mm"
equation "plasticthickness = 2 mm"
equation "d19 = box_ih + wallthickness"
equation "d20 = box_ih + wallthickness"
equation "longnotch_l = box_iw - 2 * longnotchleadin"
equation "d23 = wallthickness"
equation "nublength = box_iw / 10"
equation "longnotch_dist = longnotchleadin"
equation "nubdist = ( box_iw - 2 * cornerdim ) / 5"
equation "d52 = longnotch_dist"
equation "longnotchleadin = 10 mm"
equation "d60 = platethickness"
equation "d76 = screwd"
equation "d77 = cornerdim / 2"
equation "d78 = cornerdim / 2"
equation "d84 = box_iw - cornerdim"
equation "d85 = -( box_id - cornerdim )"
equation "top3_bezel = cornerdim * 0.3"
equation "top3_screwdist = 6 mm"
equation "d113 = top3_bezel + 2 * screwd"
equation "d114 = top3_bezel + 2 * screwd"
equation "d115 = top3_bezel + 2 * screwd"
equation "d116 = top3_bezel + 2 * screwd"
equation "d117 = box_id - top3_bezel * 2"
equation "d118 = box_iw - top3_bezel * 2"
equation "d122 = box_iw - cornerdim"
equation "d123 = -( box_iw - cornerdim )"
equation "d127 = top3_bezel"
equation "d128 = top3_bezel"
equation "d167 = screwd"
equation "d168 = plasticthickness + wallthickness + ( cornerdim / 2 )"
equation "d169 = plasticthickness + platethickness + ( cornerdim / 2 )"
equation "d179 = cornerdim / 2"
equation "d183 = wallthickness"
equation "poti_screwd = 6.5 mm"
equation "lcd_blockdisty = 2 mm"
equation "lcd_blockdistx = 0 mm"
equation "d207 = plasticthickness + wallthickness + cornerdim"
equation "d208 = cornerdim + wallthickness"
equation "d209 = screwd"
equation "d210 = cornerdim / 2"
equation "d211 = cornerdim / 2"
equation "d213 = cornerdim"
equation "d214 = cornerdim - plasticthickness"
equation "d215 = plasticthickness"
equation "d217 = plasticthickness"
equation "d219 = plasticthickness + wallthickness + cornerdim"
equation "d221 = cornerdim"
equation "d223 = screwd"
equation "d224 = cornerdim / 2"
equation "d225 = cornerdim / 2"
equation "d226 = screwd"
equation "d227 = cornerdim / 2"
equation "d228 = cornerdim / 2"
equation "d229 = screwd"
equation "d230 = cornerdim / 2"
equation "d231 = cornerdim / 2"
equation "d232 = screwd"
equation "d233 = cornerdim / 2"
equation "d234 = cornerdim / 2"
equation "d235 = -plasticthickness"
equation "d237 = -plasticthickness"
equation "d239 = -plasticthickness"
equation "d241 = -plasticthickness"
equation "d243 = screwd"
equation "d244 = cornerdim / 2"
equation "d245 = cornerdim / 2"
equation "d246 = plasticthickness"
equation "d259 = -( box_ih - cornerdim )"
equation "d260 = -( box_id - cornerdim )"
equation "d263 = box_iw - cornerdim"
equation "d264 = -( box_ih - cornerdim )"
equation "d270 = wallthickness + cornerdim / 2"
equation "d271 = wallthickness + cornerdim / 2"
equation "d272 = cornerdim / 2"
equation "d274 = cornerdim / 2"
equation "sidenub_l = box_ih / 10"
equation "d278 = wallthickness"
equation "d298 = wallthickness"
equation "d299 = wallthickness"
equation "d301 = cornerdim + wallthickness + plasticthickness"
equation "d302 = cornerdim"
equation "d303 = cornerdim + wallthickness"
equation "d304 = screwd"
equation "d305 = cornerdim / 2"
equation "d306 = cornerdim / 2"
equation "d307 = plasticthickness"
equation "d309 = plasticthickness + wallthickness + cornerdim"
equation "d311 = screwd"
equation "d312 = cornerdim / 2"
equation "d313 = cornerdim / 2"
equation "d314 = cornerdim"
equation "d315 = cornerdim"
equation "d316 = screwd"
equation "d317 = cornerdim / 2"
equation "d318 = cornerdim / 2"
equation "d319 = cornerdim - plasticthickness"
equation "d320 = cornerdim"
equation "d321 = cornerdim - plasticthickness"
equation "d322 = cornerdim - 2 * plasticthickness"
equation "d323 = plasticthickness"
equation "d324 = plasticthickness"
equation "d326 = cornerdim"
equation "d328 = cornerdim"
equation "d332 = screwd"
equation "d333 = cornerdim / 2"
equation "d334 = cornerdim / 2"
equation "d335 = -plasticthickness"
equation "d337 = screwd"
equation "d338 = plasticthickness + wallthickness + ( cornerdim / 2 )"
equation "d339 = cornerdim / 2"
equation "d342 = -plasticthickness"
equation "d348 = sidenub_l"
equation "d349 = sidenub_l"
equation "d357 = -2 * sidenub_l"
equation "d371 = box_ih + wallthickness"
equation "odd_w = 127 mm"
equation "odd_h = 13 mm"
equation "odd_d = 126 mm"
equation "odd_inset_w = 25 mm"
equation "odd_inset_d = odd_d - 90 mm"
equation "odd_inset_h = 6 mm"
equation "brk_btn_brd_d = 46 mm"
equation "brk_btn_brd_w = 35 mm"
equation "brk_aux_w = 70 mm"
equation "brk_aux_d = 26 mm"
equation "aux_d = 6 mm"
equation "aux_dist = 12 mm"
equation "brk_sata_d = 32 mm"
equation "brk_sata_w = 19 mm"
equation "port_sata_w = 6 mm"
equation "port_sata_d = 25.5 mm"
equation "port_usba_w = 13 mm"
equation "port_usba_h = 7 mm"
equation "port_usb_idist = 5.5 mm"
equation "port_usba_cornerdist = 22.5 mm"
equation "port_usba_hdmidist = 6.5 mm"
equation "port_hdmi_w = 15 mm"
equation "port_vga_h = 8 mm"
equation "port_hdmi_h = 7 mm"
equation "port_vga_wt = 16.5 mm"
equation "port_vga_wb = 13.5 mm"
equation "port_pow_d = 8 mm"
equation "port_pow_w = 21.5 mm"
equation "port_net_w = 11.5 mm"
equation "port_net_h = 13 mm"
equation "d411 = longnotchleadin"
equation "btn_pow_d = 15 mm"
equation "d418 = wallthickness"
equation "d420 = port_net_w"
equation "d421 = port_net_h"
equation "d423 = port_vga_wt"
equation "d425 = port_vga_wb"
equation "d428 = port_hdmi_h"
equation "d429 = port_hdmi_w"
equation "d430 = port_usba_h"
equation "d431 = port_usba_w"
equation "port_hdmi_vga_dist = 12.5 mm"
equation "port_net_power_dist = 4.5 mm"
equation "d438 = port_pow_d"
equation "port_net_vga_dist = 75.5 mm"
equation "fanheight = 17.5 mm"
equation "standoffheight = 20 mm"
equation "d451 = standoffheight"
equation "d457 = wallthickness"
equation "d458 = cornerdim / 2"
equation "d461 = box_iw - cornerdim"
equation "d462 = -box_ih + cornerdim"
equation "d517 = box_iw - cornerdim"
equation "d518 = -( box_id - cornerdim )"
equation "d521 = box_iw"
equation "d531 = wallthickness"
equation "d532 = wallthickness"
equation "d533 = longnotchleadin"
equation "d534 = longnotch_dist"
equation "d537 = cornerdim / 2"
equation "d538 = cornerdim / 2"
equation "d543 = wallthickness"
equation "d546 = box_iw - 2 * longnotchleadin"
equation "d572 = plasticthickness + platethickness"
equation "d592 = longnotchleadin"
equation "d593 = longnotchleadin"
equation "rift_w = 12 mm"
equation "d607 = top3_bezel + 2 * screwd"
equation "d608 = top3_bezel + 2 * screwd"
equation "d611 = lcd_boardw"
equation "d612 = -lcd_boardh"
equation "d613 = lcd_screwd"